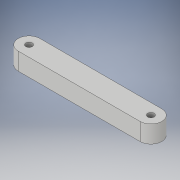
# Autodesk Inventor part: Klemme_Hebel_Entstück
Saved by Autodesk Inventor 2018 (Build 220112000, 112)
## iProperties
Created: 2018-02-02
Part Number: Klemme_Hebel_Entstück
Material: Generisch
Document SubType Name: Modeling
Designer: Julian
Density: 1 g/cm^3
Appearance: Vorgabe
Author: Julian
Autodesk Inventor part; units mm, degrees
ref_plane "YZ Plane" through (0, 0, 0) normal (1, 0, 0) x (0, 1, 0)
ref_plane "XZ Plane" through (0, 0, 0) normal (0, 1, 0) x (-1, 0, 0)
ref_plane "XY Plane" through (0, 0, 0) normal (0, 0, 1) x (1, 0, 0)
sketch "Skizze1" plane through (0, 0, 0) normal (0, 0, 1) x (1, 0, 0)
  line L0 (2.5, 0) -> (30.5, 0)
  line L1 (33, 2.5) -> (33, 2.5)
  line L2 (30.5, 5) -> (2.5, 5)
  line L3 (0, 2.5) -> (0, 2.5)
  arc A0 (2.5, 5) -> (0, 2.5) centre (2.5, 2.5) ccw
  arc A1 (0, 2.5) -> (2.5, 0) centre (2.5, 2.5) ccw
  arc A2 (33, 2.5) -> (30.5, 5) centre (30.5, 2.5) ccw
  arc A3 (30.5, 0) -> (33, 2.5) centre (30.5, 2.5) ccw
  point P0 (0, 0)
  point P1 (33, 5)
  point P2 (0, 5)
  dimension "d0" = 33
  dimension "d9" = 2.5
  constraints: 8 end point, 8 point on circle, 8 tangent, 6 point on line, 4 centre point, 3 equal radius, 2 parallel, 1 horizontal, 1 perpendicular
  measures "d0" distance of point (33, 5) point (0, 5)
  measures "d9" radius of A0
extrude "Extrusion2" add sketch "Skizze1" along normal blind 4
sketch "Skizze2" plane through (0, 0, 4) normal (0, 0, 1) x (1, 0, 0)
  arc A0 (2.5, 5) -> (2.5, 0) centre (2.5, 2.5) ccw projected
  circle A1 centre (2.5, 2.5) radius 0.75
  arc A2 (30.5, 0) -> (30.5, 5) centre (30.5, 2.5) ccw projected
  circle A3 centre (30.5, 2.5) radius 0.75
  point P0 (0, 0)
  dimension "d15" = 1.5
  dimension "d16" = 1.5
  constraints: 2 centre point, 2 coincident
  measures "d15" diameter of A1
  measures "d16" diameter of A3
extrude "Extrusion3" cut sketch "Skizze2" against normal blind 4
